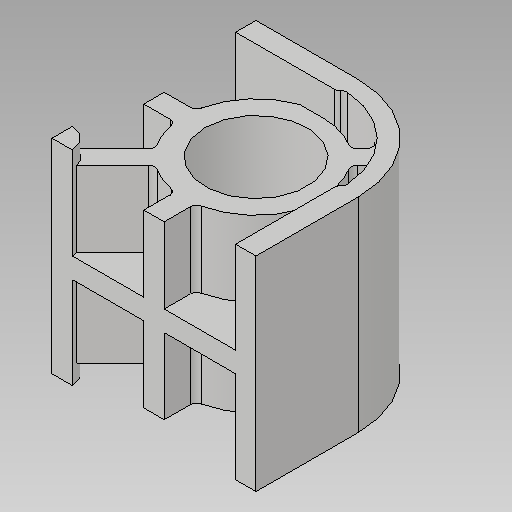
# Autodesk Inventor part: Beam_bent_base-90
Saved by Autodesk Inventor 2020 (Build 240168000, 168)
## iProperties
Created: 2019-05-05
Part Number: Beam_bent_base-90
Material: Generic
Document SubType Name: Modeling
Designer: Varga Daniel
Density: 1 g/cm^3
Appearance: Default
Author: Varga Daniel
Autodesk Inventor part; units mm, degrees
ref_plane "YZ Plane" through (0, 0, 0) normal (1, 0, 0) x (0, 1, 0)
ref_plane "XZ Plane" through (0, 0, 0) normal (0, 1, 0) x (-1, 0, 0)
ref_plane "XY Plane" through (0, 0, 0) normal (0, 0, 1) x (1, 0, 0)
derived "Base_part.ipt"
sketch "Beam_sketch" plane through (0, 0, 0) normal (0, 1, 0) x (-1, 0, 0)
  circle A0 centre (0, 0) radius 2.5
  line L0 (0, 0) -> (0, -5.5751) construction
  line L1 (3.6649, 0) -> (-4.8297, 0) construction
  arc A1 (-5, 0) -> (0, -5) centre (0, 0) ccw
  line L2 (0, -5) -> (5, -5)
  line L3 (-5, 0) -> (-5, 5)
  line L4 (-5, 5) -> (5, 5)
  line L5 (5, 5) -> (5, -5)
  line L6 (0.5, -3.4641) -> (0.5, -4)
  line L7 (-0.5, -3.2619) -> (-0.5, -4)
  line L8 (0.5, 3.4641) -> (0.5, 4)
  line L9 (-0.5, 3.4641) -> (-0.5, 4)
  line L10 (3.4641, -0.5) -> (4, -0.5)
  line L11 (3.4641, 0.5) -> (4, 0.5)
  line L12 (-3.2619, -0.5) -> (-4, -0.5)
  line L13 (-3.4641, 0.5) -> (-4, 0.5)
  line L14 (-0.5, -4) -> (4, -4)
  arc A2 (-0.5, 3.4641) -> (-3.4641, 0.5) centre (0, 0) ccw
  arc A3 (-3.2619, -0.5) -> (-0.5, -3.2619) centre (0, 0) ccw
  arc A4 (-4.1701, -0.5) -> (-0.5, -4.1701) centre (0, 0) ccw
  line L15 (4, -4) -> (4, -0.5)
  line L16 (4, -0.5) -> (4, 4)
  line L17 (4, 4) -> (0.5, 4)
  line L18 (0.5, 4) -> (-4, 4)
  line L19 (-4, 4) -> (-4, -0.5)
  arc A5 (0.5, -3.4641) -> (3.4641, -0.5) centre (0, 0) ccw
  arc A6 (3.4641, 0.5) -> (0.5, 3.4641) centre (0, 0) ccw
  line L20 (-4, -0.5) -> (-4.1701, -0.5)
  line L21 (-0.5, -4) -> (-0.5, -4.1701)
sketch "Sketch2" plane through (0, 0, 0) normal (0, 1, 0) x (-1, 0, 0)
  circle A0 centre (0, 0) radius 2.5 projected
  line L0 (0, 0) -> (0, -5.5751) construction
  line L1 (3.6649, 0) -> (-4.8297, 0) construction
  arc A1 (-5, 0) -> (0, -5) centre (0, 0) ccw
  line L2 (-5, 0) -> (-5, 5)
  line L3 (-5, 5) -> (0, 5)
  line L4 (-4, 5) -> (-4, 0)
  line L5 (5, 5) -> (-5.3684, -5.3684) construction
  line L6 (0, 0) -> (7.5921, 0) construction
  line L7 (-5, 0) -> (-4, 0) construction
  line L8 (-4, 0) -> (0, 0) construction
  line L9 (-4, 0) -> (-4.2, 0)
  arc A2 (-4.2, 0) -> (0, -4.2) centre (0, 0) ccw
  arc A3 (0, -3.5) -> (1.1662, -3.3) centre (0, 0) ccw construction
  arc A4 (-3.5, 0) -> (-2.803, -2.0959) centre (0, 0) ccw construction
  line L10 (-3.5, 0) -> (-3.3, 0) construction
  arc A5 (-3.3, 0) -> (0, -3.3) centre (0, 0) ccw
  line L11 (-3.3023, -2.5952) -> (-2.6601, -1.953)
  line L12 (0, 0) -> (0, 5) construction
  line L13 (0, 0) -> (0, -5.0311) construction
  line L14 (-2.5952, -3.3023) -> (-1.953, -2.6601)
  arc A6 (-2.0959, -2.803) -> (0, -3.5) centre (0, 0) ccw construction
  arc A7 (-2.803, -2.0959) -> (-2.0959, -2.803) centre (0, 0) ccw construction
  arc A8 (-2.803, -2.0959) -> (-2.4749, -2.4749) centre (0, 0) ccw construction
  arc A9 (-3.5, 0) -> (-2.803, -2.0959) centre (0, 0) ccw construction
  line L15 (0, -3.5) -> (0, -3.3) construction
  line L16 (0, -4.2) -> (0, -4)
  line L17 (0, -5) -> (5, -5)
  line L18 (0, -4) -> (5, -4)
  line L19 (5, 0) -> (5, -5)
  line L20 (0, 0) -> (5.9733, 0) construction
  line L21 (0, 5) -> (5, 5)
  line L22 (5, 0) -> (5, 5)
  line L23 (5, 5) -> (5, 5)
  line L24 (5, 5) -> (5, 5)
  line L25 (4, 5) -> (4, 5)
  line L26 (5, 4) -> (5, 4)
  arc A10 (4, 5) -> (5, 4) centre (5, 5) ccw
  line L27 (-0.5, 5) -> (-0.5, 3.4641)
  line L28 (0.5, 3.4641) -> (0.5, 5)
  line L29 (3.4641, -0.5) -> (5, -0.5)
  line L30 (5, 0.5) -> (3.4641, 0.5)
  line L31 (2.0959, 2.803) -> (4.2929, 5)
  line L32 (4.2929, 5) -> (5, 5)
  line L33 (5, 5) -> (5, 4.2929)
  line L34 (2.803, 2.0959) -> (5, 4.2929)
  line L35 (-3.3, 0) -> (-3.3, 1.1662)
  line L36 (0, -3.3) -> (1.1662, -3.3)
  arc A11 (-3.3, 1.1662) -> (-3.5, 0) centre (0, 0) ccw construction
  arc A12 (1.1662, -3.3) -> (-3.3, 1.1662) centre (0, 0) ccw
  dimension "d7" = 7
  dimension "d1" = 10
  dimension "d2" = 5
  dimension "d3" = 1
  dimension "d4" = 135
  dimension "d5" = 45
  dimension "d11" = 0.8
  dimension "d12" = 0.9
  dimension "d13" = 0.8
  dimension "d14" = 1
  dimension "d15" = 1
  dimension "d16" = 5
  dimension "d17" = 10
  dimension "d18" = 10
  dimension "d19" = 1
  dimension "d20" = 1
  dimension "d21" = 1
  dimension "d33" = 1
  dimension "d36" = 45
  dimension "d37" = 45
  constraints: 70 end point, 32 point on circle, 24 point on line, 14 parallel, 10 centre point, 5 coincident, 5 perpendicular, 4 tangent, 3 collinear, 1 horizontal, 28 other
  measures "d1" diameter of A1
  measures "d2" distance from line of point (0, 0) L3
  measures "d3" distance between parallel lines of L2 L4
  measures "d4" angle of L5 L6
  measures "d5" angle of L2 L5
  measures "d11" radial gap between concentric circles of A2 A1
  measures "d12" radial gap between concentric circles of A5 A2
  measures "d13" radial gap between concentric circles of A0 A5
  measures "d14" diameter of L11 L5
  measures "d15" distance between parallel lines of L18 L17
  measures "d16" distance from line of point (0, 0) L19
  measures "d17" distance from line of L21.end L2
  measures "d18" distance from line of L22.end L17
  measures "d19" distance between parallel lines of L23 L25
  measures "d20" distance between parallel lines of L28 L27
  measures "d21" distance between parallel lines of L30 L29
  measures "d33" distance between parallel lines of L34 L31
  measures "d36" angle of L32 L5
  measures "d37" angle of L5 L33
extrude "Extrusion4" add sketch "Sketch2" along normal mid plane 10 contours L2 L3 L4 L9 A2 L16 L18 L19 L17 A1 | L21 L31 A10 | A10 L34 L22 | L21 L22 L34 A10 L31
extrude "Extrusion6" add sketch "Sketch2" along normal mid plane 8.4 contours L3 L21 L28 A12 L27 | L29 A12 L30 L22 L19 | A12 L36 A5 L35 | L11 A5 L14 A2 | L31 A10 L34 A12 | L21 L22 L34 A10 L31
fillet "Fillet1" radius 0.3 8 edges at (4.2, 0, 0) (3.3, 0, 0) (0, 0, -4.2) (0, 0, -3.3) (3.3023, 0, -2.5952) (2.5952, 0, -3.3023) (2.6601, 0, -1.953) (1.953, 0, -2.6601)
extrude "Extrusion8" add sketch "Sketch2" along normal mid plane 1 contours L3 L27 A12 L35 A5 L11 A2 L9 L4 | L18 L16 A2 L14 A5 L36 A12 L29 L19 | L21 A10 L31 A12 L28 | L30 A12 L34 A10 L22 | L21 L31 A10
fillet "Fillet3" radius 0.3 12 edges at (-2.803, -2.35, 2.0959) (-3.4641, -2.35, 0.5) (-0.5, -2.35, 3.4641) (-2.0959, -2.35, 2.803) (0.5, -2.35, 3.4641) (-3.4641, -2.35, -0.5) (-3.4641, 2.35, -0.5) (-3.4641, 2.35, 0.5) (-2.803, 2.35, 2.0959) (-2.0959, 2.35, 2.803) (-0.5, 2.35, 3.4641) (0.5, 2.35, 3.4641)
fillet "Fillet4" radius 0.3 4 edges at (0, -2.75, -4) (4, -2.75, 0) (0, 2.75, -4) (4, 2.75, 0)
equation "\"d7\" = Hole_ring_diameter"
equation "\"d1\" = Outer_width"
equation "\"d2\" = 0.5 * Outer_width"
equation "\"d3\" = Wall_thickness"
equation "\"d11\" = Corner_wall_thickness"
equation "\"d12\" = Corner_gap_thickness"
equation "\"d14\" = Inner_route_thickness"
equation "\"d15\" = Wall_thickness"
equation "\"d16\" = 0.5 * Outer_width"
equation "\"d17\" = Outer_width"
equation "\"d18\" = Outer_width"
equation "\"d19\" = Wall_thickness"
equation "\"d20\" = Inner_route_thickness"
equation "\"d21\" = Inner_route_thickness"
equation "\"d33\" = Inner_route_thickness"
equation "\"d29\" = Overall_height"
equation "\"d34\" = Hole_height"
equation "\"d40\" = Inner_fillet"
equation "\"Beam_angle\" = 90deg"
equation "\"d22\" = Inner_route_thickness"
equation "\"Hole_ring_diameter\" = 7"
equation "\"Outer_width\" = 10"
equation "\"Wall_thickness\" = 1"
equation "\"Corner_wall_thickness\" = 0.8"
equation "\"Corner_gap_thickness\" = 0.9"
equation "\"Inner_route_thickness\" = 1"
equation "\"Overall_height\" = 10"
equation "\"Hole_height\" = 8.4"
equation "\"Inner_fillet\" = 0.3"
body "Solid2"
